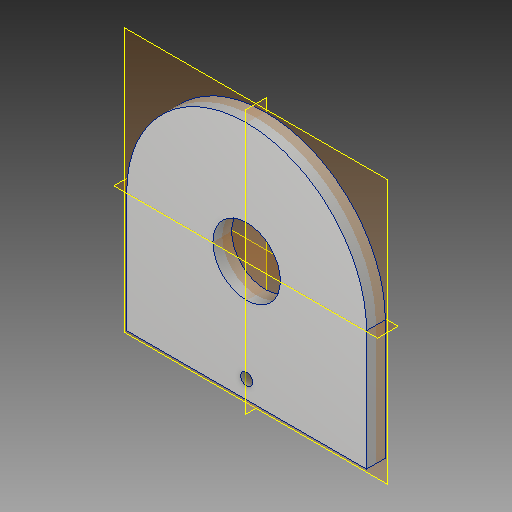
# Autodesk Inventor part: Boom Hinge
Saved by Autodesk Inventor 2019 (Build 230136000, 136)
## iProperties
Created: 2018-10-28
Part Number: Boom Hinge
Material: Aluminum 6061
Document SubType Name: Modeling
Designer: Alex Barnett
Density: 2.7 g/cm^3
Appearance: Aluminum - Flat
Author: Alex Barnett
Autodesk Inventor part; units mm, degrees
sketch "Sketch1" plane through (0, 0, 0) normal (0, 0, 1) x (1, 0, 0)
  arc A0 (50.8, 0) -> (-50.8, 0) centre (0, 0) ccw
  line L0 (50.8, 0) -> (50.8, -50.8)
  line L1 (50.8, -50.8) -> (-50.8, -50.8)
  line L2 (-50.8, -50.8) -> (-50.8, 0)
  line L3 (0, 71.12) -> (0, -71.12) projected
  dimension "d2" = 50.8
  dimension "d3" = 50.8
  dimension "d22" = 0
  constraints: 6 end point, 2 point on circle, 1 centre point, 1 parallel
  measures "d2" distance of L0.start L0.end
  measures "d3" radius of A0
  measures "d22" distance from line of L3 A0.centre
extrude "Extrusion1" add sketch "Sketch1" along normal mid plane 7.9375
sketch "Sketch2" plane through (0, 0, 3.9688) normal (0, 0, 1) x (1, 0, 0)
  point P0 (0, 0)
  point P1 (0, 0)
  constraints: 1 coincident
hole "Hole1" at (0, 0, 3.9688) direction (0, 0, -1) diameter 28.575 end through all
sketch "Sketch4" plane through (0, 0, 3.9688) normal (0, 0, 1) x (1, 0, 0)
  line L0 (-50.8, -50.8) -> (50.8, -50.8) projected
  point P0 (0, 0)
  point P1 (0, -43.18)
  dimension "d23" = 7.62
  measures "d23" distance from line of L0 point (0, -43.18)
hole "Hole3" at (0, -43.18, 3.9688) direction (0, 0, -1) diameter 5.08 end through all
body "Solid1"
